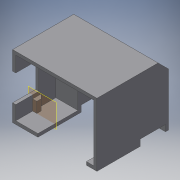
# Autodesk Inventor part: case
Saved by Autodesk Inventor 2018 (Build 220112000, 112)
## iProperties
Created: 2018-06-27
Part Number: case
Material: Generic
Document SubType Name: Modeling
Designer: erwin
Density: 1 g/cm^3
Appearance: Default
Author: erwin
Autodesk Inventor part; units mm, degrees
ref_plane "YZ Plane" through (0, 0, 0) normal (1, 0, 0) x (0, 1, 0)
ref_plane "XZ Plane" through (0, 0, 0) normal (0, 1, 0) x (-1, 0, 0)
ref_plane "XY Plane" through (0, 0, 0) normal (0, 0, 1) x (1, 0, 0)
sketch "Sketch1" plane through (0, 0, 0) normal (0, 1, 0) x (-1, 0, 0)
  line L0 (0, 0) -> (40, 0)
  line L1 (40, 0) -> (40, -30)
  line L2 (40, -30) -> (0, -30)
  line L3 (0, -30) -> (0, 0)
  dimension "d0" = 40
  dimension "d1" = 30
  constraints: 8 end point, 2 parallel, 1 horizontal, 1 perpendicular
  measures "d0" distance of L1.end L2.end
  measures "d1" distance of L0.end L1.end
extrude "Extrusion1" add sketch "Sketch1" along normal blind 30
chamfer "Chamfer1" distance 5 angle 45 2 edges at (-20, 30, 0) (-40, 30, -15)
sketch "Sketch2" plane through (0, 0, -30) normal (0, 0, -1) x (-1, 0, 0)
  line L0 (0, 28.5) -> (33, 28.5)
  line L1 (33, 28.5) -> (33, 16.5)
  line L2 (33, 16.5) -> (0, 16.5)
  line L3 (0, 16.5) -> (0, 28.5)
  line L4 (0, 30) -> (35, 30) projected
  line L5 (0, 0) -> (0, 30) projected
  dimension "d7" = 33
  dimension "d8" = 12
  dimension "d9" = 1.5
  constraints: 8 end point, 2 parallel, 1 collinear, 1 horizontal, 1 perpendicular
  measures "d7" distance of L1.end L2.end
  measures "d8" distance of L0.end L1.end
  measures "d9" distance between parallel lines of L4 L0
extrude "Extrusion2" cut sketch "Sketch2" against normal blind 3
shell "Shell1" thickness 1.5 removed faces 1 at (-13.3333, 0, -10)
sketch "Sketch3" plane through (0, 0, -27) normal (0, 0, -1) x (-1, 0, 0)
  line L0 (28, 28.5) -> (5, 28.5)
  line L1 (5, 28.5) -> (5, 16.5)
  line L2 (5, 16.5) -> (28, 16.5)
  line L3 (28, 16.5) -> (28, 28.5)
  line L4 (28, 28.5) -> (5, 16.5) construction
  line L5 (5, 28.5) -> (28, 16.5) construction
  line L6 (33, 16.5) -> (0, 16.5) projected
  line L7 (33, 28.5) -> (33, 16.5) projected
  line L8 (0, 16.5) -> (0, 28.5) projected
  point P0 (0, 0)
  point P1 (16.5, 22.5)
  dimension "d13" = 23
  dimension "d14" = 12
  dimension "d15" = 5
  dimension "d16" = 5
  constraints: 12 end point, 2 midpoint, 2 parallel, 1 collinear, 1 horizontal, 1 perpendicular
  measures "d13" distance of L2.end L1.end
  measures "d14" distance of L1.end L0.end
  measures "d15" distance between parallel lines of L7 L3
  measures "d16" distance between parallel lines of L8 L1
extrude "Extrusion3" cut sketch "Sketch3" against normal up to next
move faces "Move1" translate (0, 0, 7) faces at (-32.3333, 19.9596, -25.5)
sketch "Sketch4" plane through (0, 0, -27) normal (0, 0, -1) x (-1, 0, 0)
  line L0 (28, 28.5) -> (33, 28.5) construction
  line L1 (30.5, 28.5) -> (30.5, 16.5) construction
  line L2 (33, 16.5) -> (28, 16.5) construction
  line L3 (33, 28.5) -> (33, 16.5) construction
  line L4 (33, 22.5) -> (0, 22.5) construction
  line L5 (0, 0) -> (0, 25) construction
  line L6 (5, 16.5) -> (0, 16.5) construction
  line L7 (2.5, 16.5) -> (2.5, 28.5) construction
  point P0 (30.5, 22.5)
  point P1 (2.5, 22.5)
  constraints: 6 end point, 6 midpoint, 2 point on line, 1 perpendicular, 1 vertical
hole "Hole1" at (-30.5, 22.5, -27) at (-2.5, 22.5, -27) direction (0, 0, 1) diameter 1.5 depth 8 tip angle 118
sketch "Sketch5" plane through (-33, 16.5, -30) normal (0, 1, 0) x (1, 0, 0)
  line L0 (0, 0) -> (33, 0) projected
  line L1 (0, 0) -> (0, -3) projected
  line L2 (0, -3) -> (5, -3) projected
  line L3 (5, -3) -> (5, -11.5) projected
  line L4 (28, -11.5) -> (5, -11.5) projected
  line L5 (28, -3) -> (28, -11.5) projected
  line L6 (28, -3) -> (33, -3) projected
  line L7 (33, 0) -> (33, -3) projected
  line L8 (28, -11.5) -> (5, -11.5)
  line L9 (5, -11.5) -> (5, 0)
  line L10 (5, 0) -> (28, 0)
  line L11 (28, 0) -> (28, -11.5)
  point P0 (33, -30)
  constraints: 8 end point, 2 parallel, 1 horizontal, 1 perpendicular, 1 point on line
extrude "Extrusion4" cut sketch "Sketch5" against normal up to next contours L0 L11 L5 L4 L3 L9
sketch "Sketch6" plane through (-34.5, 15, -28.5) normal (-1, 0, 0) x (0, 0, 1)
  line L0 (0, -15) -> (0, 0) projected
  line L1 (22.8787, 13.5) -> (10, 13.5) projected
  line L2 (1.5, 13.5) -> (10, 13.5) projected
  line L3 (10, 13.5) -> (0, 13.5)
  line L4 (0, 13.5) -> (0, 0)
  line L5 (0, 0) -> (10, 0)
  line L6 (10, 0) -> (10, 13.5)
  point P0 (28.5, -15)
  constraints: 8 end point, 2 parallel, 1 horizontal, 1 perpendicular
extrude "Extrusion5" add sketch "Sketch6" along normal up to next
move faces "Move2" translate (0, -4, 0) faces at (-13.8333, 0, -0.5)
sketch "Sketch7" plane through (-40, 25, -30) normal (-1, 0, 0) x (0, 0, 1)
  line L0 (0, 0) -> (30, 0) projected
  line L1 (0, -29) -> (0, 0) projected
  line L2 (30, -29) -> (0, -29) projected
  line L3 (30, -29) -> (30, 0) projected
  line L4 (10.1397, -24) -> (23.1397, -24)
  line L5 (23.1397, -24) -> (23.1397, -18)
  line L6 (23.1397, -18) -> (10.1397, -18)
  line L7 (10.1397, -18) -> (10.1397, -24)
  line L8 (23.1397, -18) -> (10.1397, -18)
  line L9 (10.1397, -18) -> (10.1397, -29)
  line L10 (10.1397, -29) -> (23.1397, -29)
  line L11 (23.1397, -29) -> (23.1397, -18)
  point P0 (30, -25)
  dimension "d36" = 13
  dimension "d37" = 6
  dimension "d38" = 5
  constraints: 16 end point, 4 parallel, 2 horizontal, 2 perpendicular, 1 point on line
  measures "d36" distance of L6.end L5.end
  measures "d37" distance of L5.end L4.end
  measures "d38" distance between parallel lines of L2 L4
extrude "Extrusion6" cut sketch "Sketch7" against normal up to next contours L9 L4 L11 L2 | L7 L6 L5 L4
ref_plane "Work Plane1" through (-40, 4, -30) normal (0, -1, 0) x (1, 0, 0)
sketch "Sketch8" plane through (-40, 4, -30) normal (0, -1, 0) x (1, 0, 0)
  line L0 (38.5, 28.5) -> (38.5, 1.5) projected
  line L1 (38.5, 1.5) -> (35, 1.5) projected
  line L2 (35, 1.5) -> (35, 0) projected
  line L3 (35, 0) -> (40, 0) projected
  line L4 (40, 0) -> (40, 30) projected
  line L5 (40, 30) -> (0, 30) projected
  line L6 (0, 30) -> (0, 23.1397) projected
  line L7 (0, 23.1397) -> (1.5, 23.1397) projected
  line L8 (1.5, 23.1397) -> (1.5, 28.5) projected
  line L9 (1.5, 28.5) -> (38.5, 28.5) projected
  line L10 (1.5, 10.1397) -> (0, 10.1397) projected
  line L11 (0, 10.1397) -> (0, 0) projected
  line L12 (0, 0) -> (12, 0) projected
  line L13 (12, 0) -> (12, 1.5) projected
  line L14 (12, 1.5) -> (1.5, 1.5) projected
  line L15 (1.5, 1.5) -> (1.5, 10.1397) projected
  line L16 (1.5, 28.5) -> (38.5, 28.5) projected
  line L17 (38.5, 1.5) -> (36.5, 1.5)
  line L18 (36.5, 1.5) -> (36.5, 28.5)
  line L19 (36.5, 28.5) -> (38.5, 28.5)
  line L20 (38.5, 28.5) -> (38.5, 1.5)
  line L21 (12, 1.5) -> (1.5, 1.5) projected
  line L22 (1.5, 1.5) -> (3.5, 1.5)
  line L23 (3.5, 1.5) -> (3.5, 4.5)
  line L24 (3.5, 4.5) -> (1.5, 4.5)
  line L25 (1.5, 4.5) -> (1.5, 1.5)
  line L26 (1.5, 28.5) -> (3.5, 28.5)
  line L27 (3.5, 28.5) -> (3.5, 25.5)
  line L28 (3.5, 25.5) -> (1.5, 25.5)
  line L29 (1.5, 25.5) -> (1.5, 28.5)
  dimension "d42" = 2
  dimension "d43" = 2
  dimension "d44" = 3
  dimension "d45" = 2
  dimension "d46" = 3
  constraints: 24 end point, 6 parallel, 3 horizontal, 3 perpendicular, 1 point on line
  measures "d42" distance of L18.end L19.end
  measures "d43" distance of L24.end L23.end
  measures "d44" distance of L23.end L22.end
  measures "d45" distance of L27.end L28.end
  measures "d46" distance of L26.end L27.end
extrude "Extrusion7" add sketch "Sketch8" against normal blind 4 contours L0 L1 L18 L9 | L27 L28 L8 L9 | L24 L23 L14 L15
chamfer "Chamfer2" distance 2 angle 45 3 edges at (-3.5, 8, -15) (-36.5, 8, -3) (-36.5, 8, -27)
move faces "Move3" translate (0, 0, 4) faces at (-37.8333, 6, -25.5)
move faces "Move4" translate (0, 0, -1) faces at (-37.8333, 6, -4.5)
sketch "Sketch9" plane through (-40, 4, -30) normal (0, -1, 0) x (1, 0, 0)
  line L0 (5.6213, 24.3787) -> (1.5, 28.5) projected
  line L1 (38.5, 28.5) -> (38.5, 1.5) projected
  line L2 (1.5, 28.5) -> (38.5, 28.5)
  line L3 (38.5, 28.5) -> (38.5, 26.5)
  line L4 (38.5, 26.5) -> (1.5, 26.5)
  line L5 (1.5, 26.5) -> (1.5, 28.5)
  point P0 (40, 30)
  dimension "d58" = 2
  constraints: 8 end point, 2 parallel, 1 horizontal, 1 perpendicular, 1 point on line
  measures "d58" distance of L2.end L3.end
extrude "Extrusion8" add sketch "Sketch9" against normal blind 2
chamfer "Chamfer3" distance 2 angle 45 1 edges at (-20, 6, -1.5)
chamfer "Chamfer4" distance 2 angle 45 1 edges at (-5, 21.75, -18.5)
move faces "Move5" translate (0, 0, -2) faces at (-39.5, 3.3333, -19.8603) (-37.8333, 6, -21.5) (-39.5, -0.3333, -6.8603) (-37.8333, 6, -5.5)
equation "\"d15\" = d16"
body "Solid1"
